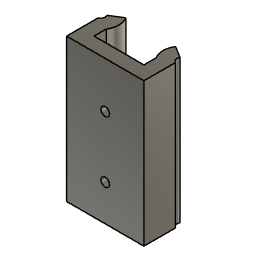
channel mount (Autodesk Fusion 360 design; units mm, degrees)
Autodesk Fusion 360 part; units mm, degrees
sketch "Sketch1" plane through (0, 0, 0) normal (0, 0, 1) x (1, 0, 0)
  line L0 (0, 0) -> (17, 0)
  line L1 (0, 0) -> (0, 4)
  line L2 (17, 0) -> (17, 4)
  arc A0 (0, 4) -> (0, 11) centre (-5.625, 7.5) ccw
  arc A1 (17, 11) -> (17, 4) centre (22.625, 7.5) ccw
  line L3 (0, 11) -> (17, 11)
  arc A2 (17.1698, 10.8943) -> (17.2, 4.0576) centre (22.625, 7.5) ccw
  line L4 (17.2, -0.2) -> (17.2, 4.0576)
  line L5 (-0.2, -0.2) -> (17.2, -0.2)
  line L6 (-0.2, -0.2) -> (-0.2, 4.0576)
  arc A3 (-0.2, 4.0576) -> (-0.1698, 10.8943) centre (-5.625, 7.5) ccw
  arc A4 (19.5472, 9.4151) -> (20, 5) centre (22.625, 7.5) ccw
  line L7 (20, -3) -> (20, 5)
  line L8 (-3, -3) -> (20, -3)
  line L9 (-3, -3) -> (-3, 5)
  arc A5 (-3, 5) -> (-2.5472, 9.4151) centre (-5.625, 7.5) ccw
  line L10 (-2.5472, 9.4151) -> (-0.1698, 10.8943)
  line L11 (19.5472, 9.4151) -> (17.1698, 10.8943)
  arc A6 (21.2453, 8.3585) -> (22, 6) centre (22.625, 7.5) ccw
  line L12 (22, -5) -> (22, 6)
  line L13 (-5, -5) -> (22, -5)
  line L14 (-5, -5) -> (-5, 6)
  arc A7 (-5, 6) -> (-4.2453, 8.3585) centre (-5.625, 7.5) ccw
  line L15 (-4.2453, 8.3585) -> (0, 11)
  line L16 (21.2453, 8.3585) -> (17, 11)
  point P0 (0, 11)
  point P1 (17, 11)
  point P2 (1, 7.5)
  point P3 (16, 7.5)
  dimension "d1" = 17
  dimension "d2" = 4
  dimension "d3" = 4
  dimension "d4" = 11
  dimension "d5" = 11
  dimension "d6" = 15
  dimension "d7" = 1
  dimension "d8" = 3.5
  dimension "d9" = 3.5
  dimension "d10" = 0.2
  dimension "d11" = 3
  dimension "d21" = -5
  constraint coincident L0.start L1.start
  constraint horizontal L0
  constraint perpendicular L0 L1
  constraint perpendicular L0 L2
  constraint coincident P2 A0
  constraint coincident P0 A0.end
  constraint coincident P3 A1
  constraint coincident P1 A1.start
  measures "d1" distance of L0.start L0.end
  measures "d2" distance of L0.start L1.end
  measures "d3" distance of L0.end L2.end
  measures "d4" distance of L0 P0
  measures "d5" distance of L0 P1
  measures "d6" distance of P2 P3
  measures "d7" horizontal distance of L2.end P3
  measures "d8" vertical distance of L2.end P3
  measures "d9" vertical distance of L1.end P2
extrude "Extrude1" add sketch "Sketch1" along normal blind 50 contours A2 L4 L5 L6 A3 A4 L7 L8 L9 A5 L10 L11 L15 L16 | A4 L7 L8 L9 A5 A6 L12 L13 L14 A7 L15 L16
sketch "Sketch4" plane through (0, -5, 0) normal (0, -1, 0) x (1, 0, 0)
  line L0 (-5, 0) -> (22, 0)
  line L1 (22, 0) -> (22, 50)
  line L2 (22, 50) -> (-5, 50)
  line L3 (-5, 50) -> (-5, 0)
  circle A0 centre (8.5, 33.9317) radius 1.5
  circle A1 centre (8.5, 12.5947) radius 1.5
  dimension "d25" = 3
  dimension "d26" = 3
  dimension "d27" = 21.337
  dimension "d28" = 13.5
  dimension "d29" = 13.5
  measures "d25" diameter of A0
  measures "d26" diameter of A1
  measures "d27" vertical distance of A0.centre A1.centre
  measures "d28" distance of L1 A0.centre
  measures "d29" distance of L1 A1.centre
extrude "Extrude3" cut sketch "Sketch4" against normal blind 4.8 contours A0 | A1
chamfer "Chamfer4" distance 2 angle 45 2 edges at (7.1015, -0.2, 33.3893) (7.1015, -0.2, 12.0523)
equation "d28 = ( 27 / 2 ) * 1 mm"
equation "d29 = ( 27 / 2 ) * 1 mm"
